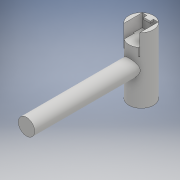
# Autodesk Inventor part: rotor1
Saved by Autodesk Inventor 2017 (Build 210142000, 142)
## iProperties
Created: 2017-08-06
Part Number: rotor1
Material: Generic
Document SubType Name: Sheet Metal
Designer: Bardo91
Density: 1 g/cm^3
Sheet Metal Rule: Default_mm
Appearance: Default
Author: Bardo91
Autodesk Inventor part; units mm, degrees
ref_plane "YZ Plane" through (0, 0, 0) normal (1, 0, 0) x (0, 1, 0)
ref_plane "XZ Plane" through (0, 0, 0) normal (0, 1, 0) x (-1, 0, 0)
ref_plane "XY Plane" through (0, 0, 0) normal (0, 0, 1) x (1, 0, 0)
sketch "Sketch1" plane through (0, 0, 0) normal (0, 0, 1) x (1, 0, 0)
  circle A0 centre (0, 0) radius 7.5
  dimension "d0" = 15
  constraints: 1 centre point, 1 coincident
  measures "d0" diameter of A0
extrude "Extrusion1" add sketch "Sketch1" along normal blind 40
sketch "Sketch2" plane through (0, 0, 40) normal (0, 0, 1) x (1, 0, 0)
  line L0 (0, 0) -> (-4.9, 0)
  line L1 (0, 0) -> (4.9, 0)
  line L2 (0, 0) -> (0, 5.5)
  line L3 (0, 5.5) -> (-4.9, 5.5)
  line L4 (-4.9, 5.5) -> (-4.9, 0)
  line L5 (0, 5.5) -> (4.9, 5.5)
  line L6 (4.9, 5.5) -> (4.9, 0)
  line L7 (-4.9, 0) -> (-4.9, -10)
  line L8 (-4.9, -10) -> (4.9, -10)
  line L9 (4.9, -10) -> (4.9, 0)
  dimension "d3" = 4.9
  dimension "d4" = 4.9
  dimension "d5" = 5.5
  dimension "d6" = 10
  constraints: 20 end point, 5 perpendicular, 2 horizontal, 2 vertical, 1 point on line
  measures "d3" distance of L0.start L0.end
  measures "d4" distance of L0.start L1.end
  measures "d5" distance of L0.start L2.end
  measures "d6" distance of L0.end L7.end
extrude "Extrusion2" cut sketch "Sketch2" against normal blind 7.9
sketch "Sketch3" plane through (0, 0, 32.1) normal (0, 0, 1) x (1, 0, 0)
  line L0 (-4.9, -5.678) -> (-4.9, 5.5) projected
  line L1 (-4.9, 5.5) -> (-4.9, 0.2)
  line L2 (-4.9, 0.2) -> (-4.4, 0.2)
  line L3 (-4.4, 0.2) -> (-4.4, -7.8)
  line L4 (-4.4, -7.8) -> (-4.9, -7.8)
  line L5 (-4.9, -7.8) -> (-4.9, 0.2)
  line L6 (4.9, 5.5) -> (4.9, -5.678) projected
  line L7 (4.9, 5.5) -> (4.9, 0.2)
  line L8 (4.9, 0.2) -> (4.4, 0.2)
  line L9 (4.4, 0.2) -> (4.4, -7.8)
  line L10 (4.4, -7.8) -> (4.9, -7.8)
  line L11 (4.9, 0.2) -> (4.9, -7.8)
  point P0 (0, 0)
  dimension "d9" = 5.3
  dimension "d10" = 0.5
  dimension "d11" = 8
  dimension "d12" = 0.5
  dimension "d13" = 5.3
  dimension "d14" = 0.5
  dimension "d15" = 8
  constraints: 20 end point, 6 point on line, 3 perpendicular, 1 horizontal
  measures "d9" distance of L0.end L1.end
  measures "d10" distance of L1.end L2.end
  measures "d11" distance of L2.end L3.end
  measures "d12" distance of L3.end L4.end
  measures "d13" distance of L6.start L7.end
  measures "d14" distance of L7.end L8.end
  measures "d15" distance of L8.end L9.end
extrude "Extrusion3" cut sketch "Sketch3" against normal blind 5
sketch "Sketch4" plane through (-4.9, 5.5, 40) normal (0, -1, 0) x (1, 0, 0)
  line L0 (12.4, 0) -> (-2.6, 0) projected
  line L1 (6.9, 0) -> (2.9, 0)
  line L2 (4.9, 0) -> (4.9, -1.2)
  line L3 (4.9, -1.2) -> (6.9, -1.2)
  line L4 (6.9, -1.2) -> (6.9, 0)
  line L5 (4.9, -1.2) -> (2.9, -1.2)
  line L6 (2.9, -1.2) -> (2.9, 0)
  point P0 (4.9, -40)
  point P1 (9.8, 0)
  point P2 (0, 0)
  dimension "d18" = 1.2
  dimension "d19" = 2
  dimension "d20" = 2
  constraints: 12 end point, 2 perpendicular, 1 collinear, 1 horizontal, 1 midpoint, 1 point on line, 1 vertical
  measures "d18" distance of L2.start L2.end
  measures "d19" distance of L2.end L3.end
  measures "d20" distance of L2.end L5.end
extrude "Extrusion4" add sketch "Sketch4" along normal blind 2
sketch "Sketch5" plane through (0, 0, 0) normal (0, 1, 0) x (-1, 0, 0)
  line L0 (-7.5, 0) -> (-7.5, 40) projected
  line L1 (-7.5, 40) -> (-7.5, 0)
  line L2 (-7.5, 20) -> (7.5, 20)
  line L3 (7.5, 0) -> (7.5, 40) projected
  circle A0 centre (0, 20) radius 5
  point P0 (0, 0)
  dimension "d23" = 10
  constraints: 4 end point, 3 midpoint, 2 point on line, 1 centre point
  measures "d23" diameter of A0
extrude "Extrusion5" add sketch "Sketch5" against normal blind 70
equation "\"BendRadius\" = Thickness"
equation "\"BendReliefWidth\" = Thickness"
equation "\"BendReliefDepth\" = 0.5 * Thickness"
equation "\"CornerReliefSize\" = 4 * Thickness"
equation "\"MinimumRemnant\" = 2 * Thickness"
equation "\"TransitionRadius\" = BendRadius"
equation "\"JacobiRadiusSize\" = BendRadius"
equation "\"GapSize\" = Thickness"
equation "\"Thickness\" = 0.5"
body "Solid1"
